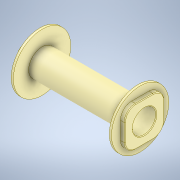
# Autodesk Inventor part: Hüllse mit Isolator
Saved by Autodesk Inventor 2021 (Build 250183000, 183)
## iProperties
Created: 2022-04-25
Part Number: Hüllse mit Isolator
Material: Nylon 6/6
Document SubType Name: Modeling
Designer: Timo
Density: 1.13 g/cm^3
Appearance: Nylon 6
Mass: 3.74667 g
Surface Area: 61.4158 cm^2
Volume: 3.31564 cm^3
Author: Timo
Autodesk Inventor part; units mm, degrees
ref_plane "YZ Plane" through (0, 0, 0) normal (1, 0, 0) x (0, 1, 0)
ref_plane "XZ Plane" through (0, 0, 0) normal (0, 1, 0) x (-1, 0, 0)
ref_plane "XY Plane" through (0, 0, 0) normal (0, 0, 1) x (1, 0, 0)
sketch "Skizze1" plane through (0, 0, 0) normal (0, 0, 1) x (1, 0, 0)
  line L0 (22.75, 13) -> (22.75, 5.3)
  line L1 (22.75, 5.3) -> (-22.75, 5.3)
  line L2 (-22.75, 5.3) -> (-22.75, 13)
  line L3 (-22.75, 0) -> (22.75, 0)
  line L4 (-22.75, 13) -> (-21.75, 13)
  line L5 (-21.75, 13) -> (-21.75, 6.1)
  line L6 (-21.75, 6.1) -> (21.75, 6.1)
  line L7 (21.75, 6.1) -> (21.75, 13)
  line L8 (21.75, 13) -> (22.75, 13)
  point P0 (0, 0)
  point P1 (0, 5.3)
  point P2 (0, 0)
  dimension "d0" = 10.6
  dimension "d2" = 45.5
  dimension "d8" = 1
  dimension "d9" = 0.8
  dimension "d10" = 26
  constraints: 18 end point, 7 perpendicular, 3 point on line, 2 midpoint, 1 coincident, 1 collinear, 1 horizontal, 1 vertical alignment
  measures "d0" diameter of L1 L3
  measures "d2" distance of L2.end L0.start
  measures "d8" distance of L2.end L4.end
  measures "d9" distance between parallel lines of L1 L6
  measures "d10" diameter of L4 L3
revolve "Umdrehung1" add sketch "Skizze1" angle 360 about axis through (-22.75, 0, 0) along (1, 0, 0)
sketch "Skizze3" plane through (22.75, 0, 0) normal (1, 0, 0) x (0, 0, -1)
  line L0 (-8.95, -8.95) -> (8.95, -8.95)
  line L1 (8.95, -8.95) -> (8.95, 8.95)
  line L2 (8.95, 8.95) -> (-8.95, 8.95)
  line L3 (-8.95, 8.95) -> (-8.95, -8.95)
  line L4 (-8.95, -8.95) -> (8.95, 8.95) construction
  line L5 (8.95, -8.95) -> (-8.95, 8.95) construction
  circle A0 centre (0, 0) radius 5.3 projected
  point P0 (0, 0)
  dimension "d11" = 17.9
  constraints: 12 end point, 2 midpoint, 2 parallel, 2 perpendicular, 1 horizontal
  measures "d11" distance of L2.end L1.end
extrude "Extrusion2" add sketch "Skizze3" along normal blind 2
fillet "Rundung2" radius 5 4 edges at (23.75, 8.95, 8.95) (23.75, 8.95, -8.95) (23.75, -8.95, 8.95) (23.75, -8.95, -8.95)
mirror "Spiegeln1" about plane through (0, 0, 0) normal (1, 0, 0) of "Extrusion2", "Rundung2"
chamfer "Fase1" distance 0.3 angle 45 4 edges at (-24.75, 0, -8.95) (-24.75, 8.95, 0) (-24.75, 0, 8.95) (-24.75, -8.95, 0)
chamfer "Fase2" distance 0.3 angle 45 4 edges at (24.75, 0, -8.95) (24.75, 8.95, 0) (24.75, 0, 8.95) (24.75, -8.95, 0)
fillet "Rundung5" radius 0.3 1 edges at (24.75, 0, 5.3)
fillet "Rundung6" radius 0.3 1 edges at (-24.75, 0, 5.3)
sketch "Skizze4" plane through (24.75, 0, 0) normal (1, 0, 0) x (0, 0, -1)
  circle A0 centre (0, 0) radius 15
  point P0 (0, 0)
  constraints: 1 centre point, 1 coincident
ref_plane "Arbeitsebene1" through (0, 0, 0) normal (1, 0, 0) x (0, 1, 0)
